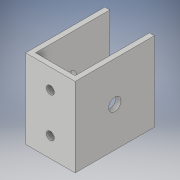
# Autodesk Inventor part: bumper attachment
Saved by Autodesk Inventor 2019 (Build 230136000, 136)
## iProperties
Created: 2018-12-26
Part Number: bumper attachment
Material: Generic
Document SubType Name: Modeling
Designer: Tiberus
Density: 1 g/cm^3
Appearance: Default
Author: Tiberus
Autodesk Inventor part; units mm, degrees
ref_plane "YZ Plane" through (0, 0, 0) normal (1, 0, 0) x (0, 1, 0)
ref_plane "XZ Plane" through (0, 0, 0) normal (0, 1, 0) x (-1, 0, 0)
ref_plane "XY Plane" through (0, 0, 0) normal (0, 0, 1) x (1, 0, 0)
sketch "Sketch1" plane through (0, 0, 0) normal (0, 0, 1) x (1, 0, 0)
  line L0 (0, 0) -> (25.4, 0)
  line L1 (25.4, 0) -> (25.4, 50.8)
  line L2 (25.4, 50.8) -> (0, 50.8)
  line L3 (0, 50.8) -> (0, 0)
  line L4 (12.7, 50.8) -> (12.7, 38.1) construction
  line L5 (12.7, 0) -> (12.7, 12.7) construction
  circle A0 centre (12.7, 38.1) radius 2.5797
  circle A1 centre (12.7, 12.7) radius 2.5797
  dimension "d0" = 25.4
  dimension "d1" = 50.8
  dimension "d2" = 12.7
  dimension "d3" = 12.7
  dimension "d4" = 5.1594
  dimension "d5" = 5.1594
  constraints: 12 end point, 2 centre point, 2 coincident, 2 midpoint, 2 parallel, 2 vertical, 1 horizontal, 1 perpendicular
  measures "d0" distance of L2.end L1.end
  measures "d1" distance of L1.end L0.end
  measures "d2" distance of L4.start L4.end
  measures "d3" distance of L5.start L5.end
  measures "d4" diameter of A0
  measures "d5" diameter of A1
extrude "Extrusion1" add sketch "Sketch1" along normal blind 3.175
sketch "Sketch2" plane through (0, 0, 0) normal (-1, 0, 0) x (0, 0, 1)
  line L0 (3.175, 0) -> (-47.625, 0)
  line L1 (-47.625, 0) -> (-47.625, 50.8)
  line L2 (-47.625, 50.8) -> (3.175, 50.8)
  line L3 (3.175, 50.8) -> (3.175, 0)
  point P0 (0, 0)
  dimension "d8" = 50.8
  dimension "d9" = 50.8
  constraints: 8 end point, 2 parallel, 1 horizontal, 1 perpendicular
  measures "d8" distance of L1.end L2.end
  measures "d9" distance of L0.end L1.end
extrude "Extrusion2" add sketch "Sketch2" along normal blind 3.175
sketch "Sketch3" plane through (25.4, 0, 0) normal (1, 0, 0) x (0, 0, -1)
  line L0 (0, 0) -> (-3.175, 0) projected
  line L1 (-3.175, 50.8) -> (47.625, 50.8) projected
  line L2 (-3.175, 0) -> (47.625, 0)
  line L3 (47.625, 0) -> (47.625, 50.8)
  line L4 (47.625, 50.8) -> (-3.175, 50.8)
  line L5 (-3.175, 50.8) -> (-3.175, 0)
  constraints: 8 end point, 2 parallel, 1 horizontal, 1 perpendicular
extrude "Extrusion3" add sketch "Sketch3" along normal blind 3.175
sketch "Sketch4" plane through (-3.175, 0, 0) normal (-1, 0, 0) x (0, 0, 1)
  point P0 (-22.225, 25.4)
hole "Hole1" at (-3.175, 25.4, -22.225) direction (1, 0, 0) diameter 8.001 depth 3.175
sketch "Sketch5" plane through (28.575, 0, 0) normal (1, 0, 0) x (0, 0, -1)
  point P0 (22.225, 25.4)
hole "Hole3" at (28.575, 25.4, -22.225) direction (-1, 0, 0) diameter 8.001 depth 3.175
body "Solid1"
